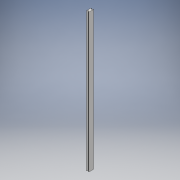
# Autodesk Inventor part: wheelRoad
Saved by Autodesk Inventor 2017 (Build 210142000, 142)
## iProperties
Created: 2016-11-26
Part Number: wheelRoad
Material: Generic
Document SubType Name: Modeling
Designer: umr
Density: 1 g/cm^3
Appearance: Default
Author: umr
Autodesk Inventor part; units mm, degrees
ref_plane "YZ Plane" through (0, 0, 0) normal (1, 0, 0) x (0, 1, 0)
ref_plane "XZ Plane" through (0, 0, 0) normal (0, 1, 0) x (-1, 0, 0)
ref_plane "XY Plane" through (0, 0, 0) normal (0, 0, 1) x (1, 0, 0)
sketch "Sketch1" plane through (0, 0, 0) normal (0, 0, 1) x (1, 0, 0)
  line L0 (0, 0) -> (50, 0)
  line L1 (50, 0) -> (50, 100)
  line L2 (50, 100) -> (0, 100)
  line L3 (0, 100) -> (0, 0)
  dimension "d0" = 50
  dimension "d1" = 100
  constraints: 8 end point, 2 parallel, 1 horizontal, 1 perpendicular
  measures "d0" distance of L2.end L1.end
  measures "d1" distance of L0.end L1.end
extrude "Extrusion1" add sketch "Sketch1" along normal blind 2900
sketch "Sketch2" plane through (0, 0, 2900) normal (0, 0, 1) x (1, 0, 0)
  line L0 (0, 0) -> (50, 0) projected
  line L1 (50, 0) -> (50, 100) projected
  line L2 (50, 100) -> (0, 100) projected
  line L3 (0, 100) -> (0, 0) projected
  line L4 (16.6667, 80) -> (33.3333, 80)
  line L5 (16.6667, 80) -> (43.3333, 80) construction
  line L6 (16.6667, 80) -> (5.1197, 100)
  line L7 (50, 100) -> (0, 100) projected
  line L8 (16.6667, 80) -> (39.7607, 80) construction
  line L9 (33.3333, 80) -> (44.8803, 100)
  line L10 (33.3333, 80) -> (56.4273, 80) construction
  line L11 (44.8803, 100) -> (5.1197, 100)
  line L12 (0, 50) -> (50, 50)
  line L13 (50, 0) -> (50, 100) projected
  line L14 (16.6667, 20) -> (33.3333, 20)
  line L15 (16.6667, 20) -> (5.1197, 0)
  line L16 (33.3333, 20) -> (44.8803, 0)
  line L17 (44.8803, 0) -> (5.1197, 0)
  dimension "d4" = 50
  dimension "d5" = 16.6667
  dimension "d6" = 100
  dimension "d7" = 20
  dimension "d8" = 16.6667
  dimension "d11" = 120
  dimension "d12" = 60
  dimension "d13" = 50
  constraints: 24 end point, 4 horizontal, 4 symmetric about line, 2 equal length, 2 midpoint, 2 point on line, 1 collinear, 1 perpendicular
  measures "d4" distance of L1.end L2.end
  measures "d5" distance of L4.start L4.end
  measures "d6" distance of L0.end L1.end
  measures "d7" distance between parallel lines of L4 L2
  measures "d8" distance from line of L1 L4.end
  measures "d11" angle of L8 L6
  measures "d12" angle of L10 L9
  measures "d13" distance between parallel lines of L0 L12
extrude "Extrusion2" cut sketch "Sketch2" against normal up to next contours L15 L14 L16 L0 | L2 L9 L4 L6
equation "\"d1\" = 2 * d0"
equation "\"d5\" = 0.333333 * d4"
equation "\"d7\" = 0.2 * d6"
equation "\"d8\" = -0.5 * d5 + 0.5 * d4"
equation "\"d13\" = 0.5 * d6"
body "Solid1"
